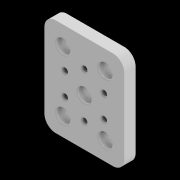
# Autodesk Inventor part: UpperArmShoulderMount
Saved by Autodesk Inventor 2020 (Build 240168000, 168)
## iProperties
Created: 2020-04-17
Part Number: UpperArmShoulderMount
Material: Generic
Document SubType Name: Sheet Metal
Designer: valer
Density: 1 g/cm^3
Sheet Metal Rule: Default
Appearance: Default
Author: valer
Autodesk Inventor part; units mm, degrees
ref_plane "YZ Plane" through (0, 0, 0) normal (1, 0, 0) x (0, 1, 0)
ref_plane "XZ Plane" through (0, 0, 0) normal (0, 1, 0) x (-1, 0, 0)
ref_plane "XY Plane" through (0, 0, 0) normal (0, 0, 1) x (1, 0, 0)
sketch "Sketch1" plane through (0, 0, 0) normal (0, 0, 1) x (1, 0, 0)
  circle A0 centre (-9.6692, -12.9185) radius 3.175
  circle A1 centre (9.3808, -12.9185) radius 3.175
  circle A2 centre (9.3808, 14.1748) radius 3.175
  circle A3 centre (-9.6692, 14.1748) radius 3.175
  line L0 (-9.6692, 14.1748) -> (9.3808, 14.1748) construction
  line L1 (9.3808, 14.1748) -> (9.3808, -12.9185) construction
  line L2 (9.3808, -12.9185) -> (-9.6692, -12.9185) construction
  line L3 (-9.6692, -12.9185) -> (-9.6692, 14.1748) construction
  line L4 (-18.1359, 22.6415) -> (17.8474, 22.6415)
  line L5 (17.8474, 22.6415) -> (17.8474, -21.3852)
  line L6 (17.8474, -21.3852) -> (-18.1359, -21.3852)
  line L7 (-18.1359, -21.3852) -> (-18.1359, 22.6415)
  circle A4 centre (0, 0) radius 10.165 construction
  circle A5 centre (0, 10.165) radius 1.27
  circle A6 centre (-8.8031, 5.0825) radius 1.27
  circle A7 centre (-8.8031, -5.0825) radius 1.27
  circle A8 centre (0, -10.165) radius 1.27
  circle A9 centre (8.8031, -5.0825) radius 1.27
  circle A10 centre (8.8031, 5.0825) radius 1.27
  dimension "d7" = 20.3299
  dimension "d0" = 8.4667
  dimension "d1" = 8.4667
  dimension "d2" = 8.4667
  dimension "d3" = 8.4667
  dimension "d4" = 6.35
  dimension "d8" = 2.54
  dimension "d11" = 360
  measures "d0" distance between parallel lines of L4 L0
  measures "d1" distance between parallel lines of L5 L1
  measures "d2" distance between parallel lines of L6 L2
  measures "d3" distance between parallel lines of L7 L3
  measures "d4" diameter of A2
  measures "d8" diameter of A5
extrude "Plate2" add sketch "Sketch1" along normal blind 5.08
fillet "Fillet1" radius 5.08 4 edges at (-18.1359, -21.3852, 2.54) (17.8474, -21.3852, 2.54) (17.8474, 22.6415, 2.54) (-18.1359, 22.6415, 2.54)
sketch "Sketch4" plane through (0, 0, 5.08) normal (0, 0, 1) x (1, 0, 0)
  point P0 (0, 0)
hole "Hole1" at (0, 0, 5.08) direction (0, 0, -1) diameter 6.35 end through all
equation "\"d18\" = Thickness"
equation "\"d5\" = Thickness"
equation "\"BendRadius\" = Thickness"
equation "\"BendReliefWidth\" = Thickness"
equation "\"BendReliefDepth\" = 0.5 * Thickness"
equation "\"CornerReliefSize\" = 4 * Thickness"
equation "\"MinimumRemnant\" = 2 * Thickness"
equation "\"TransitionRadius\" = BendRadius"
equation "\"JacobiRadiusSize\" = BendRadius"
equation "\"GapSize\" = Thickness"
equation "\"Thickness\" = 5.08"
body "Solid1"
